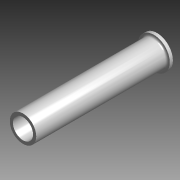
# Autodesk Inventor part: pipe
Saved by Autodesk Inventor 2015 (Build 190159000, 159)
## iProperties
Created: 2014-05-06
Part Number: pipe
Material: PVC-Piping
Document SubType Name: Modeling
Designer: Jascha
Density: 1.4 g/cm^3
Appearance: Smooth - White
Author: Jascha
Autodesk Inventor part; units mm, degrees
ref_plane "YZ Plane" through (0, 0, 0) normal (1, 0, 0) x (0, 1, 0)
ref_plane "XZ Plane" through (0, 0, 0) normal (0, 1, 0) x (-1, 0, 0)
ref_plane "XY Plane" through (0, 0, 0) normal (0, 0, 1) x (1, 0, 0)
sketch "Sketch1" plane through (0, 0, 0) normal (0, 0, 1) x (1, 0, 0)
  circle A0 centre (0, 0) radius 13.335
  circle A1 centre (0, 0) radius 10.16
  dimension "d1" = 20.32
  dimension "d5" = 26.67
  constraints: 2 centre point, 2 coincident
  measures "d1" diameter of A1
  measures "d5" diameter of A0
extrude "Extrusion1" add sketch "Sketch1" along normal blind 58.7375 and the other way blind 71.4375
sketch "Sketch2" plane through (0, 0, 0) normal (0, 1, 0) x (-1, 0, 0)
  line L0 (10.16, -71.4375) -> (10.16, 58.7375) construction
  line L1 (10.16, 58.7375) -> (13.335, 58.7375) construction
  line L2 (13.335, 58.7375) -> (13.335, -71.4375) construction
  line L3 (13.335, -71.4375) -> (10.16, -71.4375) projected
  line L4 (-10.16, 58.7375) -> (-10.16, -71.4375) construction
  line L5 (-10.16, -71.4375) -> (-13.335, -71.4375) construction
  line L6 (-13.335, -71.4375) -> (-13.335, 58.7375) construction
  line L7 (-13.335, 58.7375) -> (-10.16, 58.7375) construction
  line L8 (13.335, -71.4375) -> (13.335, -73.2656) construction
  line L9 (13.335, -73.2656) -> (16.0701, -73.2656) construction
  spline S0 degree 2 poles (13.335, -71.4375) (13.335, -73.2656) (16.0701, -73.2656) knots 1 1 1 2 2 2
  line L10 (16.0701, -73.2656) -> (16.0701, -76.4406)
  line L11 (0, -105.1255) -> (0, 86.048) projected
  spline S1 degree 5 poles (10.16, -71.4375) (10.1607, -72.3811) (10.3553, -73.3253) (10.8096, -74.2133) (12.0296, -75.5264) (13.675, -76.2036) (14.4712, -76.3698) (15.2694, -76.4406) (16.0701, -76.4406) knots 0 0 0 0 0 0 0.54113 0.54113 0.54113 1 1 1 1 1 1
  point P0 (0, 0)
  constraints: 2 end point, 2 vertical, 1 horizontal, 6 other
revolve "Revolution1" add sketch "Sketch2" angle 360 about axis through (0, 0, -10) along (0, 0, 1)
body "Solid1"
